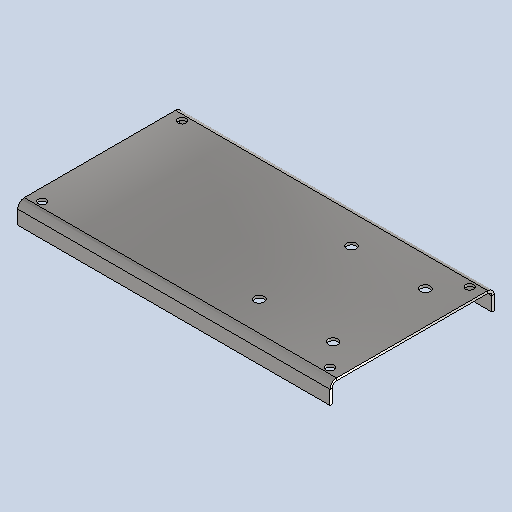
# Autodesk Inventor part: BURUN plate
Saved by Autodesk Inventor 2025 (Build 290162010, 162A)
## iProperties
Created: 2024-12-06
Part Number: BURUN plate
Material: Stainless Steel
Document SubType Name: Sheet Metal
Designer: pokla
Density: 8 g/cm^3
Sheet Metal Rule: AISI304 3mm Die 32
Appearance: Semi-Polished
Mass: 2156 g
Surface Area: 1842.06 cm^2
Volume: 269.5 cm^3
Flat Pattern Width: 23.7855 cm
Flat Pattern Length: 38 cm
Flat Pattern Area: 903.848 cm^2
Sheet Metal Width: 237,855 mm
Sheet Metal Length: 380,000 mm
Sheet Metal Area: 90384,849 mm^2
Author: pokla
Autodesk Inventor part; units mm, degrees
ref_plane "YZ Plane" through (0, 0, 0) normal (1, 0, 0) x (0, 1, 0)
ref_plane "XZ Plane" through (0, 0, 0) normal (0, 1, 0) x (-1, 0, 0)
ref_plane "XY Plane" through (0, 0, 0) normal (0, 0, 1) x (1, 0, 0)
sketch "Sketch1" plane through (0, 0, 0) normal (0, 0, 1) x (1, 0, 0)
  line L0 (-190, 100) -> (190, 100)
  line L1 (190, 100) -> (190, -100)
  line L2 (190, -100) -> (-190, -100)
  line L3 (-190, -100) -> (-190, 100)
  line L4 (-190, 100) -> (190, -100) construction
  point P0 (0, 0)
  point P1 (0, 0)
  dimension "d0" = 380
  dimension "d1" = 200
  measures "d0" distance of L0.start L0.end
  measures "d1" distance of L2.end L0.start
extrude "Plate1" add sketch "Sketch1" against normal blind 3
sketch "Sketch2" plane through (0, 0, 0) normal (0, 0, 1) x (1, 0, 0)
  line L0 (60, 56) -> (150, 56) construction
  line L1 (150, 56) -> (150, -56) construction
  line L2 (150, -56) -> (60, -56) construction
  line L3 (60, -56) -> (60, 56) construction
  line L4 (190, -100) -> (190, 100) projected
  point P0 (0, 0)
  point P1 (60, 0)
  dimension "d3" = 90
  dimension "d4" = 112
  dimension "d5" = 40
  constraints: 8 end point, 4 coincident, 2 parallel, 1 horizontal, 1 horizontal alignment, 1 midpoint, 1 perpendicular
  measures "d3" distance of L0.start L0.end
  measures "d4" distance of L0.end L1.end
  measures "d5" distance between parallel lines of L4 L1
hole "Hole1" at (60, 56, 0) at (150, 56, 0) at (60, -56, 0) at (150, -56, 0) direction (0, 0, -1) diameter 12 end through all
sketch "Sketch3" plane through (0, 0, 0) normal (0, 0, 1) x (1, 0, 0)
  line L0 (-175, 85) -> (175, 85) construction
  line L1 (175, 85) -> (175, -85) construction
  line L2 (175, -85) -> (-175, -85) construction
  line L3 (-175, -85) -> (-175, 85) construction
  line L4 (-175, 85) -> (175, -85) construction
  point P0 (0, 0)
  point P1 (0, 0)
  dimension "d14" = 170
  dimension "d15" = 350
  constraints: 10 end point, 5 coincident, 2 parallel, 1 horizontal, 1 midpoint, 1 perpendicular
  measures "d14" distance of L2.end L0.start
  measures "d15" distance of L0.start L0.end
hole "Hole2" at (-175, 85, 0) at (175, 85, 0) at (175, -85, 0) at (-175, -85, 0) direction (0, 0, -1) diameter 10 end through all
sketch "Sketch4" plane through (-190, -97, 0) normal (0, -1, 0) x (1, 0, 0)
  line L0 (380, 0) -> (0, 0)
  line L1 (0, 0) -> (0, -25)
  line L2 (0, -25) -> (380, -25)
  line L3 (380, -25) -> (380, 0)
  constraints: 6 end point, 1 horizontal, 1 perpendicular, 1 vertical
edge flange "Flange1" height 25 angle 90 thickness 3 bend radius 5 thickness toward (0, -1, 0) relief round relief width 3 relief depth 1.5 corner gap 5 corner form 0 edges at (0, -100, -3) (0, 100, -3) wall of the first edge with corners at (190, -97, 0) (-190, -97, 0) (-190, -97, -25) (190, -97, -25)
bend "Bend1"
corner "Corner1"
equation "\"d11\" = Thickness"
equation "\"d2\" = Thickness"
equation "\"d23\" = BendReliefWidth"
equation "\"d24\" = BendReliefDepth"
equation "\"d25\" = MinimumRemnant"
equation "\"d26\" = TransitionRadius"
equation "\"d29\" = BendRadius"
equation "\"d30\" = CornerReliefSize"
equation "\"d31\" = GapSize"
equation "\"d32\" = JacobiRadiusSize"
equation "\"BendReliefWidth\" = Thickness"
equation "\"BendReliefDepth\" = 0.5 * Thickness"
equation "\"CornerReliefSize\" = 4 * Thickness"
equation "\"MinimumRemnant\" = 2 * Thickness"
equation "\"TransitionRadius\" = BendRadius"
equation "\"JacobiRadiusSize\" = BendRadius"
equation "\"GapSize\" = Thickness"
equation "\"Thickness\" = 3"
equation "\"BendRadius\" = 5"
body "Solid1"
